Autodesk Inventor part; units mm, degrees
(part 2 of 2)
  arc A363 (-436.88, 400.0641) -> (-444.5, 395.6647) centre (-439.42, 395.6647) ccw
  circle A364 centre (-449.58, 413.2623) radius 15.24 construction
  line L286 (-454.66, 395.6647) -> (-454.66, 366.3353)
  arc A365 (-444.5, 366.3353) -> (-436.88, 361.9359) centre (-439.42, 366.3353) ccw
  line L287 (-444.5, 366.3353) -> (-444.5, 395.6647)
  line L288 (-411.48, 376.6006) -> (-436.88, 361.9359)
  line L289 (-436.88, 400.0641) -> (-411.48, 385.3994)
  arc A366 (-411.48, 376.6006) -> (-411.48, 385.3994) centre (-414.02, 381) ccw
  circle A367 centre (-505.46, 381) radius 15.24 construction
  arc A368 (-523.24, 376.6006) -> (-523.24, 385.3994) centre (-525.78, 381) ccw
  arc A369 (-510.54, 363.4024) -> (-518.16, 367.8018) centre (-515.62, 363.4024) ccw
  arc A370 (-548.64, 400.0641) -> (-556.26, 395.6647) centre (-551.18, 395.6647) ccw
  line L290 (-548.64, 400.0641) -> (-523.24, 385.3994)
  line L291 (-556.26, 366.3353) -> (-556.26, 395.6647)
  line L292 (-523.24, 376.6006) -> (-548.64, 361.9359)
  line L293 (-543.56, 353.1371) -> (-518.16, 367.8018)
  arc A371 (-556.26, 366.3353) -> (-548.64, 361.9359) centre (-551.18, 366.3353) ccw
  arc A372 (-543.56, 353.1371) -> (-543.56, 344.3383) centre (-541.02, 348.7377) ccw
  line L294 (-510.54, 363.4024) -> (-510.54, 334.073)
  line L295 (-518.16, 329.6736) -> (-543.56, 344.3383)
  arc A373 (-548.64, 335.5394) -> (-556.26, 331.14) centre (-551.18, 331.14) ccw
  line L296 (-548.64, 335.5394) -> (-523.24, 320.8747)
  arc A374 (-523.24, 312.0759) -> (-523.24, 320.8747) centre (-525.78, 316.4753) ccw
  line L297 (-556.26, 301.8106) -> (-556.26, 331.14)
  line L298 (-523.24, 312.0759) -> (-548.64, 297.4112)
  line L299 (-543.56, 288.6124) -> (-518.16, 303.2771)
  arc A375 (-543.56, 288.6124) -> (-543.56, 279.8136) centre (-541.02, 284.213) ccw
  line L300 (-518.16, 265.1489) -> (-543.56, 279.8136)
  arc A376 (-518.16, 265.1489) -> (-510.54, 269.5483) centre (-515.62, 269.5483) ccw
  line L301 (-510.54, 298.8777) -> (-510.54, 269.5483)
  arc A377 (-467.36, 279.8136) -> (-467.36, 288.6124) centre (-469.9, 284.213) ccw
  arc A378 (-462.28, 297.4112) -> (-454.66, 301.8106) centre (-459.74, 301.8106) ccw
  arc A379 (-492.76, 303.2771) -> (-500.38, 298.8777) centre (-495.3, 298.8777) ccw
  line L302 (-492.76, 303.2771) -> (-467.36, 288.6124)
  line L303 (-500.38, 269.5483) -> (-500.38, 298.8777)
  line L304 (-467.36, 279.8136) -> (-492.76, 265.1489)
  arc A380 (-500.38, 269.5483) -> (-492.76, 265.1489) centre (-495.3, 269.5483) ccw
  line L305 (-462.28, 361.9359) -> (-487.68, 376.6006)
  line L306 (-500.38, 334.073) -> (-500.38, 363.4024)
  arc A381 (-492.76, 367.8018) -> (-500.38, 363.4024) centre (-495.3, 363.4024) ccw
  line L307 (-492.76, 367.8018) -> (-467.36, 353.1371)
  line L308 (-477.52, 359.003) -> (-472.44, 367.8018)
  arc A382 (-492.76, 367.8018) -> (-500.38, 363.4024) centre (-495.3, 363.4024) ccw
  arc A383 (-492.76, 367.8018) -> (-500.38, 363.4024) centre (-495.3, 363.4024) ccw
  line L309 (-492.76, 367.8018) -> (-467.36, 353.1371)
  line L310 (-492.76, 367.8018) -> (-467.36, 353.1371)
  line L311 (-500.38, 334.073) -> (-500.38, 363.4024)
  line L312 (-500.38, 334.073) -> (-500.38, 363.4024)
  line L313 (-467.36, 344.3383) -> (-492.76, 329.6736)
  line L314 (-487.68, 320.8747) -> (-462.28, 335.5394)
  line L315 (-487.68, 320.8747) -> (-462.28, 335.5394)
  line L316 (-467.36, 344.3383) -> (-492.76, 329.6736)
  line L317 (-467.36, 344.3383) -> (-492.76, 329.6736)
  arc A384 (-487.68, 320.8747) -> (-487.68, 312.0759) centre (-485.14, 316.4753) ccw
  arc A385 (-500.38, 334.073) -> (-492.76, 329.6736) centre (-495.3, 334.073) ccw
  circle A386 centre (-337.82, 477.787) radius 15.24 construction
  circle A387 centre (-579.12, 493.9182) radius 17.8404 construction
  point P0 (0, 0)
  point P1 (-430.9533, 381)
  point P2 (-403.86, 381)
  point P3 (-444.5, 357.5365)
  point P4 (-444.5, 404.4635)
  point P5 (-398.78, 372.2012)
  point P6 (-398.78, 325.2742)
  point P7 (-439.42, 348.7377)
  point P8 (-388.62, 372.2012)
  point P9 (-347.98, 348.7377)
  point P10 (-388.62, 325.2742)
  point P11 (-383.54, 381)
  point P12 (-342.9, 404.4635)
  point P13 (-342.9, 357.5365)
  point P14 (-388.62, 389.7988)
  point P15 (-388.62, 436.7258)
  point P16 (-347.98, 413.2623)
  point P17 (-398.78, 389.7988)
  point P18 (-439.42, 413.2623)
  point P19 (-398.78, 436.7258)
  point P20 (-388.62, 348.7377)
  point P21 (-398.78, 348.7377)
  point P22 (-441.96, 361.9359)
  point P23 (-454.66, 357.5365)
  point P24 (-495.3, 381)
  point P25 (-457.2, 361.9359)
  point P26 (-454.66, 404.4635)
  point P27 (-454.66, 383.9329)
  point P28 (-457.2, 400.0641)
  point P29 (-459.74, 348.7377)
  point P30 (-500.38, 325.2742)
  point P31 (-464.82, 348.7377)
  point P32 (-500.38, 372.2012)
  point P33 (-482.6, 361.9359)
  point P34 (-497.84, 367.8018)
  point P35 (-454.66, 339.9388)
  point P36 (-454.66, 293.0118)
  point P37 (-457.2, 335.5394)
  point P38 (-495.3, 316.4753)
  point P39 (-477.52, 326.7406)
  point P40 (-490.22, 316.4753)
  point P41 (-444.5, 339.9388)
  point P42 (-403.86, 316.4753)
  point P43 (-441.96, 335.5394)
  point P44 (-444.5, 293.0118)
  point P45 (-444.5, 313.5424)
  point P46 (-441.96, 297.4112)
  point P47 (-439.42, 348.7377)
  point P48 (-398.78, 372.2012)
  point P49 (-434.34, 348.7377)
  point P50 (-398.78, 325.2742)
  point P51 (-416.56, 335.5394)
  point P52 (-401.32, 329.6736)
  point P53 (-398.78, 260.7495)
  point P54 (-398.78, 307.6765)
  point P55 (-439.42, 284.213)
  point P56 (-416.56, 271.0148)
  point P57 (-401.32, 265.1489)
  point P58 (-434.34, 284.213)
  point P59 (-347.98, 284.213)
  point P60 (-388.62, 307.6765)
  point P61 (-388.62, 260.7495)
  point P62 (-365.76, 273.9477)
  point P63 (-353.06, 284.213)
  point P64 (-386.08, 265.1489)
  point P65 (-342.9, 339.9388)
  point P66 (-383.54, 316.4753)
  point P67 (-342.9, 293.0118)
  point P68 (-342.9, 319.4083)
  point P69 (-345.44, 335.5394)
  point P70 (-345.44, 297.4112)
  point P71 (-388.62, 372.2012)
  point P72 (-388.62, 325.2742)
  point P73 (-347.98, 348.7377)
  point P74 (-370.84, 361.9359)
  point P75 (-386.08, 367.8018)
  point P76 (-353.06, 348.7377)
  point P77 (-439.42, 348.7377)
  point P78 (-398.78, 325.2742)
  point P79 (-398.78, 372.2012)
  point P80 (-421.64, 359.003)
  point P81 (-434.34, 348.7377)
  point P82 (-401.32, 367.8018)
  point P83 (-398.78, 325.2742)
  point P84 (-439.42, 348.7377)
  point P85 (-434.34, 348.7377)
  point P86 (-444.5, 357.5365)
  point P87 (-287.02, 389.7988)
  point P88 (-292.1, 381)
  point P89 (-297.18, 381)
  point P90 (-421.64, 359.003)
  point P91 (-398.78, 372.2012)
  point P92 (-401.32, 367.8018)
  point P93 (-403.86, 381)
  point P94 (-444.5, 404.4635)
  point P95 (-439.42, 477.787)
  point P96 (-398.78, 501.2505)
  point P97 (-388.62, 501.2505)
  point P98 (-398.78, 454.3235)
  point P99 (-388.62, 454.3235)
  point P100 (-347.98, 477.787)
  point P101 (-398.78, 436.7258)
  point P102 (-388.62, 436.7258)
  point P103 (-388.62, 436.7258)
  point P104 (-388.62, 436.7258)
  point P105 (-383.54, 445.5247)
  point P106 (-403.86, 445.5247)
  point P107 (-383.54, 445.5247)
  point P108 (-342.9, 468.9882)
  point P109 (-342.9, 422.0612)
  point P110 (-342.9, 468.9882)
  point P111 (-342.9, 422.0612)
  point P112 (-378.46, 445.5247)
  point P113 (-365.76, 455.79)
  point P114 (-347.98, 413.2623)
  point P115 (-332.74, 422.0612)
  point P116 (-327.66, 413.2623)
  point P117 (-347.98, 413.2623)
  point P118 (-353.06, 413.2623)
  point P119 (-386.08, 432.3264)
  point P120 (-412.3267, 413.2623)
  point P121 (-439.42, 413.2623)
  point P122 (-398.78, 389.7988)
  point P123 (-401.32, 394.1982)
  point P124 (-444.5, 422.0612)
  point P125 (-408.94, 381)
  point P126 (-426.72, 394.1982)
  point P127 (-441.96, 400.0641)
  point P128 (-444.5, 468.9882)
  point P129 (-388.62, 389.7988)
  point P130 (-388.62, 389.7988)
  point P131 (-386.08, 394.1982)
  point P132 (-386.08, 394.1982)
  point P133 (-388.62, 389.7988)
  point P134 (-388.62, 372.2012)
  point P135 (-383.54, 381)
  point P136 (-386.08, 367.8018)
  point P137 (-378.46, 381)
  point P138 (-388.62, 325.2742)
  point P139 (-388.62, 345.8047)
  point P140 (-386.08, 329.6736)
  point P141 (-360.68, 367.8018)
  point P142 (-347.98, 348.7377)
  point P143 (-342.9, 357.5365)
  point P144 (-345.44, 361.9359)
  point P145 (-342.9, 404.4635)
  point P146 (-332.74, 357.5365)
  point P147 (-330.2, 361.9359)
  point P148 (-332.74, 404.4635)
  point P149 (-309.88, 370.7347)
  point P150 (-289.56, 394.1982)
  point P151 (-287.02, 416.1953)
  point P152 (-287.02, 436.7258)
  point P153 (-289.56, 432.3264)
  point P154 (-330.2, 464.5888)
  point P155 (-332.74, 468.9882)
  point P156 (-345.44, 464.5888)
  point P157 (-292.1, 445.5247)
  point P158 (-314.96, 458.7229)
  point P159 (-297.18, 445.5247)
  point P160 (-388.62, 410.3294)
  point P161 (-347.98, 413.2623)
  point P162 (-365.76, 402.997)
  point P163 (-368.3, 424.9941)
  point P164 (-363.22, 433.7929)
  point P165 (-347.98, 413.2623)
  point P166 (-388.62, 389.7988)
  point P167 (-386.08, 394.1982)
  point P168 (-398.78, 389.7988)
  point P169 (-347.98, 542.3117)
  point P170 (-342.9, 533.5128)
  point P171 (-345.44, 529.1134)
  point P172 (-388.62, 410.3294)
  point P173 (-388.62, 436.7258)
  point P174 (-386.08, 432.3264)
  point P175 (-398.78, 436.7258)
  point P176 (-439.42, 413.2623)
  point P177 (-500.38, 454.3235)
  point P178 (-500.38, 501.2505)
  point P179 (-495.3, 510.0493)
  point P180 (-459.74, 477.787)
  point P181 (-454.66, 486.5858)
  point P182 (-454.66, 533.5128)
  point P183 (-444.5, 468.9882)
  point P184 (-439.42, 477.787)
  point P185 (-439.42, 477.787)
  point P186 (-439.42, 477.787)
  point P187 (-444.5, 486.5858)
  point P188 (-454.66, 468.9882)
  point P189 (-444.5, 486.5858)
  point P190 (-444.5, 533.5128)
  point P191 (-403.86, 510.0493)
  point P192 (-444.5, 533.5128)
  point P193 (-403.86, 510.0493)
  point P194 (-441.96, 490.9852)
  point P195 (-444.5, 507.1164)
  point P196 (-398.78, 501.2505)
  point P197 (-398.78, 518.8482)
  point P198 (-388.62, 518.8482)
  point P199 (-398.78, 501.2505)
  dimension "d68" = 25.4
  dimension "d76" = 5.08
  dimension "d77" = 25.4
  dimension "d80" = 360
  dimension "d82" = 10.16
  dimension "d85" = 360
  dimension "d89" = 360
  dimension "d93" = 360
  constraints: 648 point on line, 616 end point, 578 point on circle, 314 centre point, 15 tangent, 10 coincident, 6 equal radius, 5 horizontal alignment, 2 midpoint, 1 equal length, 1 horizontal, 1 perpendicular, 1 vertical, 1 vertical alignment, 2454 other
  measures "d68" distance between parallel lines of L6 L10
  measures "d76" radius of A69
  measures "d77" horizontal distance of A69.centre A70.centre
  measures "d82" distance of point (-388.62, 348.738) point (-398.78, 348.738)
body "Solid1"
